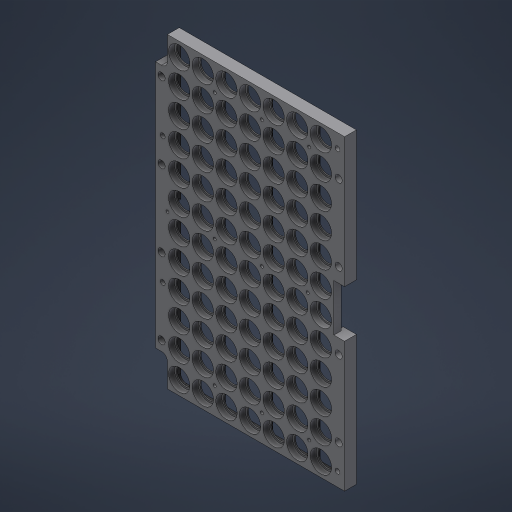
# Autodesk Inventor part: Platte2
Saved by Autodesk Inventor 2024.3 (Build 283343010, 343A)
## iProperties
Created: 2025-03-19
Part Number: Platte2
Material: Generisch
Document SubType Name: Modeling
Designer: David Lill
Density: 1 g/cm^3
Appearance: Vorgabe
Author: David Lill
Autodesk Inventor part; units mm, degrees
ref_plane "YZ Plane" through (0, 0, 0) normal (1, 0, 0) x (0, 1, 0)
ref_plane "XZ Plane" through (0, 0, 0) normal (0, 1, 0) x (-1, 0, 0)
ref_plane "XY Plane" through (0, 0, 0) normal (0, 0, 1) x (1, 0, 0)
sketch "Skizze1" plane through (0, 0, 0) normal (0, 1, 0) x (-1, 0, 0)
  line L0 (160, 0) -> (0, 0)
  line L1 (0, 0) -> (0, -260)
  line L2 (0, -260) -> (160, -260)
  line L3 (160, -260) -> (160, 0)
  circle A0 centre (140, -11.75) radius 9
  circle A1 centre (140, -54.75) radius 9
  circle A2 centre (140, -97.75) radius 9
  circle A3 centre (140, -140.75) radius 9
  circle A4 centre (140, -183.75) radius 9
  circle A5 centre (140, -226.75) radius 9
  circle A6 centre (120, -11.75) radius 9
  circle A7 centre (120, -54.75) radius 9
  circle A8 centre (120, -97.75) radius 9
  circle A9 centre (120, -140.75) radius 9
  circle A10 centre (120, -183.75) radius 9
  circle A11 centre (120, -226.75) radius 9
  circle A12 centre (100, -11.75) radius 9
  circle A13 centre (100, -54.75) radius 9
  circle A14 centre (100, -97.75) radius 9
  circle A15 centre (100, -140.75) radius 9
  circle A16 centre (100, -183.75) radius 9
  circle A17 centre (100, -226.75) radius 9
  circle A18 centre (80, -11.75) radius 9
  circle A19 centre (80, -54.75) radius 9
  circle A20 centre (80, -97.75) radius 9
  circle A21 centre (80, -140.75) radius 9
  circle A22 centre (80, -183.75) radius 9
  circle A23 centre (80, -226.75) radius 9
  circle A24 centre (60, -11.75) radius 9
  circle A25 centre (60, -54.75) radius 9
  circle A26 centre (60, -97.75) radius 9
  circle A27 centre (60, -140.75) radius 9
  circle A28 centre (60, -183.75) radius 9
  circle A29 centre (60, -226.75) radius 9
  circle A30 centre (40, -11.75) radius 9
  circle A31 centre (40, -54.75) radius 9
  circle A32 centre (40, -97.75) radius 9
  circle A33 centre (40, -140.75) radius 9
  circle A34 centre (40, -183.75) radius 9
  circle A35 centre (40, -226.75) radius 9
  circle A36 centre (20, -11.75) radius 9
  circle A37 centre (20, -54.75) radius 9
  circle A38 centre (20, -97.75) radius 9
  circle A39 centre (20, -140.75) radius 9
  circle A40 centre (20, -183.75) radius 9
  circle A41 centre (20, -226.75) radius 9
  circle A42 centre (140, -33.25) radius 9
  circle A43 centre (120, -33.25) radius 9
  circle A44 centre (100, -33.25) radius 9
  circle A45 centre (80, -33.25) radius 9
  circle A46 centre (60, -33.25) radius 9
  circle A47 centre (40, -33.25) radius 9
  circle A48 centre (20, -33.25) radius 9
  circle A49 centre (140, -76.25) radius 9
  circle A50 centre (120, -76.25) radius 9
  circle A51 centre (100, -76.25) radius 9
  circle A52 centre (80, -76.25) radius 9
  circle A53 centre (60, -76.25) radius 9
  circle A54 centre (40, -76.25) radius 9
  circle A55 centre (20, -76.25) radius 9
  circle A56 centre (140, -119.25) radius 9
  circle A57 centre (120, -119.25) radius 9
  circle A58 centre (100, -119.25) radius 9
  circle A59 centre (80, -119.25) radius 9
  circle A60 centre (60, -119.25) radius 9
  circle A61 centre (40, -119.25) radius 9
  circle A62 centre (20, -119.25) radius 9
  circle A63 centre (140, -162.25) radius 9
  circle A64 centre (120, -162.25) radius 9
  circle A65 centre (100, -162.25) radius 9
  circle A66 centre (80, -162.25) radius 9
  circle A67 centre (60, -162.25) radius 9
  circle A68 centre (40, -162.25) radius 9
  circle A69 centre (20, -162.25) radius 9
  circle A70 centre (140, -205.25) radius 9
  circle A71 centre (120, -205.25) radius 9
  circle A72 centre (100, -205.25) radius 9
  circle A73 centre (80, -205.25) radius 9
  circle A74 centre (60, -205.25) radius 9
  circle A75 centre (40, -205.25) radius 9
  circle A76 centre (20, -205.25) radius 9
  circle A77 centre (140, -248.25) radius 9
  circle A78 centre (120, -248.25) radius 9
  circle A79 centre (100, -248.25) radius 9
  circle A80 centre (80, -248.25) radius 9
  circle A81 centre (60, -248.25) radius 9
  circle A82 centre (40, -248.25) radius 9
  circle A83 centre (20, -248.25) radius 9
  line L4 (-20, 0) -> (-187, 0)
  line L5 (-207, 0) -> (-374, 0)
  circle A84 centre (140, -11.75) radius 7.5
  line L6 (155.379, -44.5989) -> (146.379, -44.5989)
  line L7 (157, -62) -> (150, -62)
  line L8 (150, -62) -> (150, -69)
  line L9 (150, -69) -> (157, -69)
  line L10 (157, -69) -> (157, -62)
  line L11 (160, -130) -> (0, -130) construction
  line L12 (157, -198) -> (150, -198)
  line L13 (150, -198) -> (150, -191)
  line L14 (150, -191) -> (157, -191)
  line L15 (157, -191) -> (157, -198)
  point P0 (80, 0)
  point P1 (153.5, -62)
  point P2 (157, -65.5)
  dimension "d0" = 160
  dimension "d1" = 260
  dimension "d4" = 18
  dimension "d7" = 43
  dimension "d10" = 20
  dimension "d16" = 21.5
  dimension "d21" = 20
  dimension "d24" = 43
  dimension "d69" = 15
  dimension "d80" = 0
  dimension "d127" = 10.75
  dimension "d129" = 7
  dimension "d130" = 7
  dimension "d132" = 3
  dimension "d134" = 10.75
  constraints: 85 centre point, 32 end point, 14 coincident, 6 horizontal, 5 midpoint, 4 parallel, 4 symmetric about line, 2 horizontal alignment, 2 perpendicular, 2 vertical, 1 equal radius, 1 vertical alignment, 164 other
  measures "d0" distance of L0.start L0.end
  measures "d1" distance of L2.end L0.start
  measures "d4" diameter of A0
  measures "d7" distance of A0.centre A1.centre
  measures "d10" distance of A0.centre A6.centre
  measures "d16" distance of A42.centre A0.centre
  measures "d21" distance of A42.centre A43.centre
  measures "d24" distance of A42.centre A49.centre
  measures "d69" diameter of A84
  measures "d80" horizontal distance of A0.centre A42.centre
  measures "d127" vertical distance of L11.start point (140, -119.25)
  measures "d129" distance of L9.end L8.end
  measures "d130" distance of L8.end L7.end
  measures "d132" distance between parallel lines of L3 L10
  measures "d134" vertical distance of point (140, -76.25) point (157, -65.5)
extrude "Extrusion1" add sketch "Skizze1" along normal blind 10 contours L3 L2 L1 L0 | A0 | A1 | A2 | A3 | A4 | A5 | A6 | A7 | A8 | A9 | A10 | A11 | A12 | A13 | A14 | A15 | A16 | A17 | A18 | A19 | A20 | A21 | A22 | A23 | A24 | A25 | A26 | A27 | A28 | A29 | A30 | A31 | A32 | A33 | A34 | A35 | A36 | A37 | A38 | A39 | A40 | A41 | A42 | A43 | A44 | A45 | A46 | A47 | A48 | A49 | A50 | A51 | A52 | A53 | A54 | A55 | A56 | A57 | A58 | A59 | A60 | A61 | A62 | A63 | A64 | A65 | A66 | A67 | A68 | A69 | A70 | A71 | A72 | A73 | A74 | A75 | A76 | A77 | A78 | A79 | A80 | A81 | A82 | A83 | A84 | L10 L9 L8 L7 | L12 L13 L14 L15
hole "Bohrung1" at (-140, 0, -11.75) at (-140, 0, -33.25) at (-140, 0, -54.75) at (-140, 0, -76.25) at (-140, 0, -97.75) at (-140, 0, -119.25) at (-140, 0, -140.75) at (-140, 0, -162.25) at (-140, 0, -183.75) at (-140, 0, -205.25) at (-140, 0, -226.75) at (-140, 0, -248.25) direction (0, 1, 0) diameter 15 end through all counterbore diameter 18 counterbore depth 5
pattern_linear "Rechteckige Anordnung1" count 7 spacing 20 along (1, 0, 0) of "Bohrung1"
sketch "Skizze2" plane through (0, 10, 0) normal (0, 1, 0) x (1, 0, 0)
  circle A0 centre (-20, 226.75) radius 9 projected
  circle A1 centre (-20, 248.25) radius 9 projected
  circle A2 centre (-20, 205.25) radius 9 projected
  circle A3 centre (-20, 162.25) radius 9 projected
  circle A4 centre (-20, 119.25) radius 9 projected
  circle A5 centre (-20, 33.25) radius 9 projected
  circle A6 centre (-20, 11.75) radius 9
  circle A7 centre (-20, 54.75) radius 9 projected
  circle A8 centre (-20, 97.75) radius 9 projected
  circle A9 centre (-20, 140.75) radius 9 projected
  circle A10 centre (-20, 183.75) radius 9 projected
  circle A11 centre (-40, 226.75) radius 9 projected
  circle A12 centre (-40, 248.25) radius 9 projected
  circle A13 centre (-40, 205.25) radius 9 projected
  circle A14 centre (-40, 162.25) radius 9 projected
  circle A15 centre (-40, 119.25) radius 9 projected
  circle A16 centre (-40, 76.25) radius 9 projected
  circle A17 centre (-40, 33.25) radius 9 projected
  circle A18 centre (-40, 11.75) radius 9 projected
  circle A19 centre (-40, 54.75) radius 9 projected
  circle A20 centre (-40, 97.75) radius 9 projected
  circle A21 centre (-40, 140.75) radius 9 projected
  circle A22 centre (-40, 183.75) radius 9 projected
  circle A23 centre (-60, 226.75) radius 9 projected
  circle A24 centre (-60, 248.25) radius 9 projected
  circle A25 centre (-60, 205.25) radius 9 projected
  circle A26 centre (-60, 162.25) radius 9 projected
  circle A27 centre (-60, 119.25) radius 9 projected
  circle A28 centre (-60, 76.25) radius 9 projected
  circle A29 centre (-60, 33.25) radius 9 projected
  circle A30 centre (-60, 11.75) radius 9 projected
  circle A31 centre (-60, 54.75) radius 9 projected
  circle A32 centre (-60, 97.75) radius 9 projected
  circle A33 centre (-60, 140.75) radius 9 projected
  circle A34 centre (-60, 183.75) radius 9 projected
  circle A35 centre (-80, 226.75) radius 9 projected
  circle A36 centre (-80, 248.25) radius 9 projected
  circle A37 centre (-80, 205.25) radius 9 projected
  circle A38 centre (-80, 162.25) radius 9 projected
  circle A39 centre (-80, 119.25) radius 9 projected
  circle A40 centre (-80, 76.25) radius 9 projected
  circle A41 centre (-80, 33.25) radius 9 projected
  circle A42 centre (-80, 11.75) radius 9 projected
  circle A43 centre (-80, 54.75) radius 9 projected
  circle A44 centre (-80, 97.75) radius 9 projected
  circle A45 centre (-80, 140.75) radius 9 projected
  circle A46 centre (-80, 183.75) radius 9 projected
  circle A47 centre (-100, 226.75) radius 9 projected
  circle A48 centre (-100, 248.25) radius 9 projected
  circle A49 centre (-100, 205.25) radius 9 projected
  circle A50 centre (-100, 162.25) radius 9 projected
  circle A51 centre (-100, 119.25) radius 9 projected
  circle A52 centre (-100, 76.25) radius 9 projected
  circle A53 centre (-100, 33.25) radius 9 projected
  circle A54 centre (-100, 11.75) radius 9 projected
  circle A55 centre (-100, 54.75) radius 9 projected
  circle A56 centre (-100, 97.75) radius 9 projected
  circle A57 centre (-100, 140.75) radius 9 projected
  circle A58 centre (-100, 183.75) radius 9 projected
  circle A59 centre (-120, 226.75) radius 9 projected
  circle A60 centre (-120, 248.25) radius 9 projected
  circle A61 centre (-120, 205.25) radius 9 projected
  circle A62 centre (-120, 162.25) radius 9 projected
  circle A63 centre (-120, 119.25) radius 9 projected
  circle A64 centre (-120, 76.25) radius 9 projected
  circle A65 centre (-120, 33.25) radius 9 projected
  circle A66 centre (-120, 11.75) radius 9 projected
  circle A67 centre (-120, 54.75) radius 9 projected
  circle A68 centre (-120, 97.75) radius 9 projected
  circle A69 centre (-120, 140.75) radius 9 projected
  circle A70 centre (-120, 183.75) radius 9 projected
  circle A71 centre (-140, 226.75) radius 9 projected
  circle A72 centre (-140, 183.75) radius 9 projected
  circle A73 centre (-140, 140.75) radius 9 projected
  circle A74 centre (-140, 97.75) radius 9 projected
  circle A75 centre (-140, 54.75) radius 9 projected
  circle A76 centre (-140, 11.75) radius 9 projected
  circle A77 centre (-140, 33.25) radius 9 projected
  circle A78 centre (-140, 76.25) radius 9 projected
  circle A79 centre (-140, 119.25) radius 9 projected
  circle A80 centre (-140, 162.25) radius 9 projected
  circle A81 centre (-140, 205.25) radius 9 projected
  circle A82 centre (-140, 248.25) radius 9 projected
  line L0 (0, 0) -> (0, 260) projected
  line L1 (-160, 0) -> (0, 0) projected
  line L2 (-160, 260) -> (-160, 0) projected
  line L3 (0, 260) -> (-160, 260) projected
  line L4 (-160, 0) -> (0, 0) projected
  line L5 (-150, 0) -> (-150, 55)
  arc A83 (-150, 55) -> (-155, 60) centre (-155, 55) ccw
  line L6 (-155, 60) -> (-160, 60)
  line L7 (-160, 260) -> (-160, 0) projected
  line L8 (-160, 0) -> (0, 0) projected
  line L9 (0, 0) -> (0, 260) projected
  line L10 (-160, 260) -> (-160, 0) projected
  line L11 (0, 260) -> (-160, 260) projected
  line L12 (-160, 25) -> (-155, 25)
  arc A84 (-150, 20) -> (-155, 25) centre (-155, 20) ccw
  line L13 (0, 130) -> (-160, 130)
  line L14 (-150, 260) -> (-150, 205)
  arc A85 (-155, 200) -> (-150, 205) centre (-155, 205) ccw
  line L15 (-155, 200) -> (-160, 200)
  line L16 (-160, 235) -> (-155, 235)
  arc A86 (-155, 235) -> (-150, 240) centre (-155, 240) ccw
  circle A87 centre (-20, 11.75) radius 9 projected
  line L17 (-143.0414, 85.25) -> (-151, 85.25)
  arc A88 (-151, 85.25) -> (-151, 67.25) centre (-151, 76.25) ccw
  line L18 (-151, 67.25) -> (-143.0414, 67.25)
  arc A89 (-143.0414, 85.25) -> (-143.0414, 67.25) centre (-140, 76.25) ccw
  line L19 (-143.0414, 174.75) -> (-151, 174.75)
  arc A90 (-151, 192.75) -> (-151, 174.75) centre (-151, 183.75) ccw
  line L20 (-151, 192.75) -> (-143.0414, 192.75)
  arc A91 (-143.0414, 192.75) -> (-143.0414, 174.75) centre (-140, 183.75) ccw
  circle A92 centre (-154, 76.25) radius 4
  circle A93 centre (-154, 183.75) radius 4
  line L21 (-80, 260) -> (-80, 0)
  line L22 (0, 232.75) -> (-3, 232.75)
  arc A94 (-3, 232.75) -> (-3, 220.75) centre (-3, 226.75) ccw
  line L23 (-3, 220.75) -> (0, 220.75)
  line L24 (0, 168.25) -> (-3, 168.25)
  arc A95 (-3, 168.25) -> (-3, 156.25) centre (-3, 162.25) ccw
  line L25 (-3, 156.25) -> (0, 156.25)
  line L26 (-160, 168.25) -> (-157, 168.25)
  arc A96 (-157, 156.25) -> (-157, 168.25) centre (-157, 162.25) ccw
  line L27 (-157, 156.25) -> (-160, 156.25)
  line L28 (0, 27.25) -> (-3, 27.25)
  arc A97 (-3, 39.25) -> (-3, 27.25) centre (-3, 33.25) ccw
  line L29 (-3, 39.25) -> (0, 39.25)
  line L30 (0, 91.75) -> (-3, 91.75)
  arc A98 (-3, 103.75) -> (-3, 91.75) centre (-3, 97.75) ccw
  line L31 (-3, 103.75) -> (0, 103.75)
  arc A99 (-157, 91.75) -> (-157, 103.75) centre (-157, 97.75) ccw
  line L32 (-160, 91.75) -> (-157, 91.75)
  line L33 (-157, 103.75) -> (-160, 103.75)
  line L34 (-16.9586, 20.75) -> (-9, 20.75)
  arc A100 (-9, 2.75) -> (-9, 20.75) centre (-9, 11.75) ccw
  line L35 (-9, 2.75) -> (-16.9586, 2.75)
  arc A101 (-16.9586, 2.75) -> (-16.9586, 20.75) centre (-20, 11.75) ccw
  circle A102 centre (-6, 11.75) radius 4
  arc A103 (-9, 239.25) -> (-9, 257.25) centre (-9, 248.25) ccw
  line L36 (-9, 257.25) -> (-16.9586, 257.25)
  arc A104 (-16.9586, 239.25) -> (-16.9586, 257.25) centre (-20, 248.25) ccw
  line L37 (-16.9586, 239.25) -> (-9, 239.25)
  circle A105 centre (-6, 248.25) radius 4
  line L38 (-160, 232.75) -> (-157, 232.75)
  arc A106 (-157, 220.75) -> (-157, 232.75) centre (-157, 226.75) ccw
  line L39 (-157, 220.75) -> (-160, 220.75)
  arc A107 (-157, 27.25) -> (-157, 39.25) centre (-157, 33.25) ccw
  line L40 (-160, 27.25) -> (-157, 27.25)
  line L41 (-157, 39.25) -> (-160, 39.25)
  line L42 (-11, 199.5) -> (-3, 199.5)
  line L43 (-3, 199.5) -> (-3, 179.5)
  line L44 (-3, 179.5) -> (-11, 179.5)
  line L45 (-11, 179.5) -> (-11, 199.5)
  line L46 (-11, 60.5) -> (-3, 60.5)
  line L47 (-3, 60.5) -> (-3, 80.5)
  line L48 (-3, 80.5) -> (-11, 80.5)
  line L49 (-11, 80.5) -> (-11, 60.5)
  line L50 (-156.36, 69) -> (-149.36, 69)
  line L51 (-149.36, 69) -> (-149.36, 62)
  line L52 (-149.36, 62) -> (-156.36, 62)
  line L53 (-156.36, 62) -> (-156.36, 69)
  line L54 (-156.36, 191) -> (-149.36, 191)
  line L55 (-149.36, 191) -> (-149.36, 198)
  line L56 (-149.36, 198) -> (-156.36, 198)
  line L57 (-156.36, 198) -> (-156.36, 191)
  point P0 (-160, 60)
  point P1 (0, 130)
  point P2 (-150, 260)
  point P3 (-160, 200)
  point P4 (-160, 235)
  point P5 (-160, 25)
  point P6 (0, 27.25)
  point P7 (0, 39.25)
  point P8 (0, 103.75)
  point P9 (-5, 226.75)
  point P10 (-5, 162.25)
  point P11 (-5, 33.25)
  point P12 (-5, 97.75)
  point P13 (-155, 226.75)
  point P14 (-155, 162.25)
  point P15 (-155, 97.75)
  point P16 (-155, 33.25)
  point P17 (-7, 199.5)
  point P18 (-7, 179.5)
  point P19 (-3, 189.5)
  point P20 (-11, 189.5)
  point P21 (-152.86, 69)
  point P22 (-149.36, 65.5)
  dimension "d83" = 10
  dimension "d84" = 5
  dimension "d85" = 60
  dimension "d101" = 25
  dimension "d119" = 8
  dimension "d121" = 6
  dimension "d124" = 33.25
  dimension "d125" = 64.5
  dimension "d126" = 6
  dimension "d135" = 9.5
  dimension "d136" = 3
  dimension "d142" = 6
  dimension "d143" = 5
  dimension "d144" = 5
  dimension "d160" = 8
  dimension "d162" = 3
  dimension "d165" = 20
  dimension "d166" = 5.75
  dimension "d169" = 7
  dimension "d170" = 7
  dimension "d171" = 3.64
  dimension "d172" = 10.75
  constraints: 107 centre point, 96 end point, 68 symmetric about line, 40 point on circle, 14 tangent, 11 midpoint, 9 point on line, 7 horizontal, 7 parallel, 7 perpendicular, 6 coincident, 6 equal radius, 6 horizontal alignment, 2 vertical, 2 vertical alignment, 1 concentric, 14 other
  measures "d83" distance between parallel lines of L2 L5
  measures "d84" radius of A83
  measures "d85" distance between parallel lines of L6 L4
  measures "d101" distance between parallel lines of L4 L12
  measures "d119" diameter of A92
  measures "d121" distance from line of L2 A92.centre
  measures "d124" distance from line of L11 point (-3, 226.75)
  measures "d125" distance of point (-3, 226.75) point (-3, 162.25)
  measures "d126" radius of A94
  measures "d135" radius of A89
  measures "d136" distance from line of L0 point (-3, 226.75)
  measures "d142" distance from line of L9 A102.centre
  measures "d143" distance from line of L0 point (-5, 226.75)
  measures "d144" distance from line of L0 point (-5, 162.25)
  measures "d160" distance of point (-3, 189.5) point (-11, 189.5)
  measures "d162" distance from line of L9 L42.end
  measures "d165" distance of L42.end L43.end
  measures "d166" distance from line of A2.centre L42
  measures "d169" distance from line of L52 point (-152.86, 69)
  measures "d170" distance of L50.start L50.end
  measures "d171" distance between parallel lines of L10 L53
  measures "d172" vertical distance of A89.centre point (-149.36, 65.5)
extrude "Extrusion2" cut sketch "Skizze2" against normal blind 10 contours L14 A86 L16 L2 L3 | L12 A84 L5 L1 L2
sketch "Skizze3" plane through (0, 10, 0) normal (0, 1, 0) x (1, 0, 0)
  point P0 (0, 0)
sketch "Skizze4" plane through (0, 10, 0) normal (0, 1, 0) x (1, 0, 0)
  line L0 (-150, 0) -> (0, 0) projected
  line L1 (0, 260) -> (-150, 260) projected
  line L2 (-16.25, 258) -> (-23.75, 258)
  line L3 (-23.75, 2) -> (-16.25, 2)
  arc A0 (-16.25, 2) -> (-11.25, 7) centre (-16.25, 7) ccw
  line L4 (-11.25, 7) -> (-11.25, 253)
  arc A1 (-11.25, 253) -> (-16.25, 258) centre (-16.25, 253) ccw
  circle A2 centre (-20, 248.25) radius 7.5 projected
  arc A3 (-148.75, 7) -> (-143.75, 2) centre (-143.75, 7) ccw
  arc A4 (-143.75, 258) -> (-148.75, 253) centre (-143.75, 253) ccw
  line L5 (-148.75, 253) -> (-148.75, 7)
  circle A5 centre (-140, 248.25) radius 7.5 projected
  line L6 (0, 0) -> (0, 260) projected
  line L7 (0, 0) -> (0, 260) projected
  line L8 (0, 0) -> (0, 260) projected
  line L9 (0, 0) -> (0, 260) projected
  line L10 (0, 0) -> (0, 260) projected
  line L11 (-150, 260) -> (-150, 240) projected
  arc A6 (-155, 235) -> (-150, 240) centre (-155, 240) ccw projected
  line L12 (-155, 235) -> (-160, 235) projected
  line L13 (-160, 235) -> (-160, 25) projected
  line L14 (-160, 235) -> (-160, 25) projected
  line L15 (-160, 235) -> (-160, 25) projected
  line L16 (-160, 235) -> (-160, 25) projected
  line L17 (-150, 20) -> (-150, 0) projected
  arc A7 (-150, 20) -> (-155, 25) centre (-155, 20) ccw projected
  line L18 (-160, 25) -> (-155, 25) projected
  line L19 (-160, 235) -> (-160, 25) projected
  line L20 (-11.25, 110) -> (0, 110)
  line L21 (-11.25, 150) -> (0, 150)
  line L22 (-143.75, 2) -> (-150, 2)
  line L23 (-143.75, 258) -> (-150, 258)
  arc A8 (-153.75, 62) -> (-148.75, 67) centre (-153.75, 67) ccw
  line L24 (-153.75, 62) -> (-160, 62)
  line L25 (-160, 198) -> (-153.75, 198)
  arc A9 (-148.75, 193) -> (-153.75, 198) centre (-153.75, 193) ccw
  line L26 (-143.75, 258) -> (-116.25, 258)
  line L27 (-111.25, 253) -> (-111.25, 136)
  line L28 (-116.25, 131) -> (-143.75, 131)
  line L29 (-148.75, 136) -> (-148.75, 253)
  arc A10 (-143.75, 258) -> (-148.75, 253) centre (-143.75, 253) ccw
  arc A11 (-111.25, 253) -> (-116.25, 258) centre (-116.25, 253) ccw
  arc A12 (-148.75, 136) -> (-143.75, 131) centre (-143.75, 136) ccw
  arc A13 (-116.25, 131) -> (-111.25, 136) centre (-116.25, 136) ccw
  line L30 (-71.25, 253) -> (-71.25, 136)
  arc A14 (-71.25, 253) -> (-76.25, 258) centre (-76.25, 253) ccw
  arc A15 (-103.75, 258) -> (-108.75, 253) centre (-103.75, 253) ccw
  line L31 (-76.25, 131) -> (-103.75, 131)
  arc A16 (-108.75, 136) -> (-103.75, 131) centre (-103.75, 136) ccw
  arc A17 (-76.25, 131) -> (-71.25, 136) centre (-76.25, 136) ccw
  line L32 (-103.75, 258) -> (-76.25, 258)
  line L33 (-108.75, 136) -> (-108.75, 253)
  line L34 (-31.25, 253) -> (-31.25, 136)
  arc A18 (-31.25, 253) -> (-36.25, 258) centre (-36.25, 253) ccw
  arc A19 (-63.75, 258) -> (-68.75, 253) centre (-63.75, 253) ccw
  line L35 (-36.25, 131) -> (-63.75, 131)
  arc A20 (-68.75, 136) -> (-63.75, 131) centre (-63.75, 136) ccw
  arc A21 (-36.25, 131) -> (-31.25, 136) centre (-36.25, 136) ccw
  line L36 (-63.75, 258) -> (-36.25, 258)
  line L37 (-68.75, 136) -> (-68.75, 253)
  line L38 (-111.25, 124) -> (-111.25, 7)
  arc A22 (-111.25, 124) -> (-116.25, 129) centre (-116.25, 124) ccw
  arc A23 (-143.75, 129) -> (-148.75, 124) centre (-143.75, 124) ccw
  line L39 (-116.25, 2) -> (-143.75, 2)
  arc A24 (-148.75, 7) -> (-143.75, 2) centre (-143.75, 7) ccw
  arc A25 (-116.25, 2) -> (-111.25, 7) centre (-116.25, 7) ccw
  line L40 (-143.75, 129) -> (-116.25, 129)
  line L41 (-148.75, 7) -> (-148.75, 124)
  line L42 (-71.25, 124) -> (-71.25, 7)
  arc A26 (-71.25, 124) -> (-76.25, 129) centre (-76.25, 124) ccw
  arc A27 (-103.75, 129) -> (-108.75, 124) centre (-103.75, 124) ccw
  line L43 (-76.25, 2) -> (-103.75, 2)
  arc A28 (-108.75, 7) -> (-103.75, 2) centre (-103.75, 7) ccw
  arc A29 (-76.25, 2) -> (-71.25, 7) centre (-76.25, 7) ccw
  line L44 (-103.75, 129) -> (-76.25, 129)
  line L45 (-108.75, 7) -> (-108.75, 124)
  line L46 (-31.25, 124) -> (-31.25, 7)
  arc A30 (-31.25, 124) -> (-36.25, 129) centre (-36.25, 124) ccw
  arc A31 (-63.75, 129) -> (-68.75, 124) centre (-63.75, 124) ccw
  line L47 (-36.25, 2) -> (-63.75, 2)
  arc A32 (-68.75, 7) -> (-63.75, 2) centre (-63.75, 7) ccw
  arc A33 (-36.25, 2) -> (-31.25, 7) centre (-36.25, 7) ccw
  line L48 (-63.75, 129) -> (-36.25, 129)
  line L49 (-68.75, 7) -> (-68.75, 124)
  line L50 (-28.75, 253) -> (-28.75, 121.2242)
  line L51 (-28.75, 121.2242) -> (-28.75, 7)
  arc A34 (-23.75, 258) -> (-28.75, 253) centre (-23.75, 253) ccw
  arc A35 (-28.75, 7) -> (-23.75, 2) centre (-23.75, 7) ccw
  line L52 (-143.75, 2) -> (-16.25, 2)
  line L53 (-143.75, 258) -> (-16.25, 258)
  line L54 (-9, 150) -> (-9, 110)
  circle A36 centre (-110, 130) radius 3.6639
  circle A37 centre (-70, 130) radius 3.6639
  arc A38 (-150.875, 132.8696) -> (-150.875, 127.1304) centre (-150, 130) ccw
  arc A39 (-148.75, 124.2609) -> (-150.875, 127.1304) centre (-151.75, 124.2609) ccw
  arc A40 (-150.875, 132.8696) -> (-148.75, 135.7391) centre (-151.75, 135.7391) ccw
  circle A41 centre (-110, 22.5073) radius 2.5
  circle A42 centre (-70, 22.5073) radius 2.5
  circle A43 centre (-30, 22.5073) radius 2.5
  circle A44 centre (-30, 237.4927) radius 2.5
  circle A45 centre (-70, 237.4927) radius 2.5
  circle A46 centre (-110, 237.4927) radius 2.5
  point P0 (-150, 20)
  point P1 (-150, 252)
  point P2 (-150, 8)
  point P3 (-11.25, 130)
  point P4 (0, 33.25)
  point P5 (-160, 162.25)
  point P6 (-111.25, 131)
  point P7 (-111.25, 258)
  point P8 (-148.75, 131)
  point P9 (-71.25, 258)
  point P10 (-71.25, 131)
  point P11 (-108.75, 131)
  point P12 (-31.25, 258)
  point P13 (-31.25, 131)
  point P14 (-68.75, 131)
  point P15 (-111.25, 129)
  point P16 (-111.25, 2)
  point P17 (-148.75, 2)
  point P18 (-71.25, 129)
  point P19 (-71.25, 2)
  point P20 (-108.75, 2)
  point P21 (-31.25, 129)
  point P22 (-31.25, 2)
  point P23 (-68.75, 2)
  point P24 (-28.75, 2)
  point P25 (-143.75, 2)
  point P26 (-36.25, 258)
  point P27 (-63.75, 258)
  point P28 (-76.25, 258)
  point P29 (-148.75, 124)
  point P30 (-143.75, 129)
  point P31 (-108.75, 124)
  point P32 (-103.75, 129)
  point P33 (-68.75, 124)
  point P34 (-63.75, 129)
  point P35 (-36.25, 258)
  point P36 (-68.75, 253)
  point P37 (-63.75, 258)
  point P38 (-76.25, 258)
  point P39 (-108.75, 253)
  point P40 (-31.25, 130)
  point P41 (-150, 130)
  point P42 (-148.75, 135.3118)
  point P43 (-148.75, 124.2609)
  point P44 (-148.75, 135.7391)
  point P45 (-31.25, 20.3422)
  point P46 (-31.25, 24.6723)
  point P47 (-28.75, 20.3422)
  point P48 (-28.75, 24.6723)
  point P49 (-68.75, 24.6723)
  point P50 (-68.75, 20.3422)
  point P51 (-71.25, 20.3422)
  point P52 (-71.25, 24.6723)
  point P53 (-111.25, 20.3422)
  point P54 (-111.25, 24.6723)
  point P55 (-108.75, 20.3422)
  point P56 (-108.75, 24.6723)
  point P57 (-31.25, 235.3277)
  point P58 (-31.25, 239.6578)
  point P59 (-28.75, 235.3277)
  point P60 (-28.75, 239.6578)
  point P61 (-71.25, 235.3277)
  point P62 (-71.25, 239.6578)
  point P63 (-68.75, 235.3277)
  point P64 (-68.75, 239.6578)
  point P65 (-111.25, 235.3277)
  point P66 (-111.25, 239.6578)
  point P67 (-108.75, 235.3277)
  point P68 (-108.75, 239.6578)
  dimension "d180" = 2
  dimension "d181" = 2
  dimension "d182" = 5
  dimension "d184" = 8.75
  dimension "d185" = 8.75
  dimension "d190" = 40
  dimension "d191" = 20
  dimension "d195" = 60
  dimension "d196" = 60
  dimension "d222" = 37.5
  dimension "d223" = 127
  dimension "d224" = 5
  dimension "d227" = 40
  dimension "d230" = 129
  dimension "d233" = 0
  dimension "d234" = 0
  dimension "d235" = 2.5
  dimension "d236" = 5
  dimension "d237" = 5
  dimension "d240" = 9
  dimension "d248" = 1.25
  dimension "d251" = 40
  dimension "d252" = 107.5
  dimension "d253" = 107.5
  dimension "d254" = 3
  dimension "d255" = 2.5
  dimension "d256" = 3
  dimension "d257" = 5
  constraints: 78 end point, 70 point on circle, 56 point on line, 43 centre point, 34 tangent, 14 equal radius, 9 coincident, 7 perpendicular, 6 horizontal alignment, 5 vertical alignment, 4 horizontal, 4 parallel, 3 vertical, 1 midpoint, 125 other
  measures "d180" distance between parallel lines of L1 L2
  measures "d181" distance between parallel lines of L0 L3
  measures "d182" radius of A1
  measures "d184" distance from line of L5 A5.centre
  measures "d185" distance from line of A2.centre L4
  measures "d190" distance between parallel lines of L21 L20
  measures "d191" distance from line of point (-11.25, 130) L20
  measures "d195" distance between parallel lines of L24 L22
  measures "d196" distance between parallel lines of L25 L23
  measures "d222" distance of point (-111.25, 131) point (-148.75, 131)
  measures "d223" distance of point (-111.25, 258) point (-111.25, 131)
  measures "d224" radius of A10
  measures "d227" distance of L27.start L30.start
  measures "d230" distance of L27.start L38.start
  measures "d233" distance between parallel lines of L2 L26
  measures "d234" distance between parallel lines of L5 L29
  measures "d235" distance between parallel lines of L51 L46
  measures "d236" radius of A34
  measures "d237" radius of A35
  measures "d240" distance between parallel lines of L54 L6
  measures "d248" distance from line of L51 point (-30, 22.507)
  measures "d251" distance of point (-110, 130) point (-150, 130)
  measures "d252" distance of point (-31.25, 130) point (-30, 22.507)
  measures "d253" distance of point (-30, 237.493) point (-31.25, 130)
  measures "d254" radius of A38
  measures "d255" distance from line of L50 point (-31.25, 130)
  measures "d256" radius of A40
  measures "d257" diameter of A41
extrude "Extrusion6" cut sketch "Skizze4" against normal blind 4 contours A3 L5 A23 L40 A22 L38 A41 A25 L39 | L20 L4 L21 L54 | A25 L38 A41 L45 A28 L52 | L4 A0 L3 A35 L51 A43 L50 A44 A34 L2 A1 | A28 L45 A41 A27 L44 A26 L42 A42 A29 L43 | L5 A12 L28 A13 A36 A22 L40 A23 | A41 L38 | L38 A41 L45 | A29 L42 A42 L49 A32 L52 | A39 A38 A40 L5 | L38 A22 A36 A27 L45 A41 | L45 A41 | A32 L49 A42 A31 L48 A30 L46 A43 A33 L47 | L26 A11 L27 A46 A13 L28 A12 L5 A4 | L52 A33 L46 A43 L51 A35 | A42 L42 | L42 A42 L49 | L53 A15 L33 A46 L27 A11 | A34 L50 A44 L34 A18 L53 | A36 | L42 A26 A37 A31 L49 A42 | L49 A42 | L32 A14 L30 A45 A17 L31 A16 L33 A46 A15 | A18 L34 A44 A21 L35 A20 L37 A45 A19 L36 | A43 L46 L51 | L51 A43 | A13 L27 A46 L33 A16 A36 | A36 A16 L31 A17 A37 A26 L44 A27 | A43 L46 | A46 L33 L27 | L27 A46 | L53 A19 L37 A45 L30 A14 | A44 L50 | L50 A44 L34 | A43 L46 A30 L48 A31 A37 A20 L35 A21 L34 A44 L50 L51 | A37 | A46 L33 | L34 A44 | A17 L30 A45 L37 A20 A37 | A45 L37 L30 | L30 A45 | A45 L37 | A5
extrude "Extrusion7" cut sketch "Skizze4" along normal through all both and the other way through all contours L20 L54 L21 L6
sketch "Skizze5" plane through (0, 0, 0) normal (0, -1, 0) x (1, 0, 0)
  point P0 (0, 0)
  point P1 (-5, -33.25)
  point P2 (-5, -97.75)
  point P3 (-5, -162.25)
  point P4 (-5, -226.75)
  point P5 (-155, -226.75)
  point P6 (-155, -162.25)
  point P7 (-155, -97.75)
  point P8 (-155, -33.25)
hole "Bohrung5" at (-5, 0, -33.25) at (-5, 0, -97.75) at (-5, 0, -162.25) at (-5, 0, -226.75) at (-155, 0, -226.75) at (-155, 0, -162.25) at (-155, 0, -97.75) at (-155, 0, -33.25) direction (0, 1, 0) diameter 4 end through all counterbore diameter 6 counterbore depth 5
hole "Bohrung6" at (-6, 10, -11.75) at (-6, 10, -248.25) at (-154, 10, -183.75) at (-154, 10, -76.25) direction (0, -1, 0) diameter 4 end through all counterbore diameter 6 counterbore depth 5
extrude "Extrusion9" add sketch "Skizze4" along normal blind 2 from surface at -4 contours A25 L38 A41 L45 A28 L52 | L5 A12 L28 A13 A36 A22 L40 A23 | A41 L38 | L38 A41 L45 | A29 L42 A42 L49 A32 L52 | A39 A38 A40 L5 | L38 A22 A36 A27 L45 A41 | L45 A41 | L52 A33 L46 A43 L51 A35 | A42 L42 | L42 A42 L49 | L53 A15 L33 A46 L27 A11 | A34 L50 A44 L34 A18 L53 | A36 | L42 A26 A37 A31 L49 A42 | L49 A42 | A43 L46 L51 | L51 A43 | A13 L27 A46 L33 A16 A36 | A36 A16 L31 A17 A37 A26 L44 A27 | A43 L46 | A46 L33 L27 | L27 A46 | L53 A19 L37 A45 L30 A14 | A44 L50 | L50 A44 L34 | A43 L46 A30 L48 A31 A37 A20 L35 A21 L34 A44 L50 L51 | A37 | A46 L33 | L34 A44 | A17 L30 A45 L37 A20 A37 | A45 L37 L30 | L30 A45 | A45 L37
hole "Bohrung7" at (-110, 10, -130) at (-70, 10, -130) at (-31.25, 10, -130) at (-150, 10, -130) at (-110, 10, -237.4927) at (-70, 10, -237.4927) at (-30, 10, -237.4927) at (-30, 10, -22.5073) at (-70, 10, -22.5073) at (-110, 10, -22.5073) direction (0, -1, 0) diameter 2.5 end through all
fillet "Rundung3" radius 3 24 edges at (-68.75, 7, -24.6723) (-68.75, 7, -20.3422) (-71.25, 7, -20.3422) (-71.25, 7, -24.6723) (-28.75, 7, -24.6723) (-28.75, 7, -20.3422) (-31.25, 7, -20.3422) (-31.25, 7, -24.6723) (-108.75, 7, -20.3422) (-108.75, 7, -24.6723) (-111.25, 7, -20.3422) (-111.25, 7, -24.6723) (-28.75, 7, -239.6578) (-31.25, 7, -239.6578) (-31.25, 7, -235.3277) (-28.75, 7, -235.3277) (-68.75, 7, -239.6578) (-71.25, 7, -239.6578) (-71.25, 7, -235.3277) (-68.75, 7, -235.3277) (-108.75, 7, -239.6578) (-111.25, 7, -235.3277) (-108.75, 7, -235.3277) (-111.25, 7, -239.6578)
equation "\"d16\" = 0.5 * d7"
equation "\"d21\" = d10"
equation "\"d24\" = d7"
